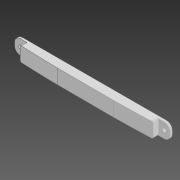
# Autodesk Inventor part: MidiPickup
Saved by Autodesk Inventor 2020 (Build 240168000, 168)
## iProperties
Created: 2022-11-12
Part Number: MidiPickup
Material: Generic
Document SubType Name: Modeling
Designer: valer
Density: 1 g/cm^3
Appearance: Default
Author: valer
Autodesk Inventor part; units mm, degrees
ref_plane "YZ Plane" through (0, 0, 0) normal (1, 0, 0) x (0, 1, 0)
ref_plane "XZ Plane" through (0, 0, 0) normal (0, 1, 0) x (-1, 0, 0)
ref_plane "XY Plane" through (0, 0, 0) normal (0, 0, 1) x (1, 0, 0)
sketch "Base" plane through (0, 0, 0) normal (0, 0, 1) x (1, 0, 0)
  line L0 (-64, -0.5) -> (64, -0.5) construction
  circle A0 centre (-64, -0.5) radius 1.5
  circle A1 centre (64, -0.5) radius 1.5
  line L1 (-64, 6) -> (64, 6)
  line L2 (69, 1) -> (69, -2)
  line L3 (64, -7) -> (-64, -7)
  line L4 (-69, -2) -> (-69, 1)
  line L5 (-59, 6) -> (-59, -7) construction
  line L6 (59, 6) -> (59, -7) construction
  arc A2 (-64, 6) -> (-69, 1) centre (-64, 1) ccw
  arc A3 (-69, -2) -> (-64, -7) centre (-64, -2) ccw
  arc A4 (69, 1) -> (64, 6) centre (64, 1) ccw
  arc A5 (64, -7) -> (69, -2) centre (64, -2) ccw
  point P0 (0, 0)
  dimension "d0" = 128
  dimension "d1" = 3
  dimension "d2" = 3
  dimension "d3" = 5
  dimension "d4" = 5
  dimension "d5" = 5
  dimension "d6" = 5
  dimension "d7" = 5
  dimension "d8" = 6.5
  dimension "d9" = 6.5
  constraints: 14 end point, 8 point on circle, 8 tangent, 6 centre point, 4 point on line, 3 equal radius, 2 coincident, 2 horizontal, 2 parallel, 2 vertical, 1 perpendicular
  measures "d0" distance of L0.start L0.end
  measures "d1" diameter of A0
  measures "d2" diameter of A1
  measures "d3" distance from line of L4 L0.start
  measures "d4" distance from line of L2 L0.end
  measures "d5" distance from line of L0.start L5
  measures "d6" distance from line of L0.end L6
  measures "d7" radius of A2
  measures "d8" distance between parallel lines of L1 L0
  measures "d9" distance between parallel lines of L3 L0
extrude "BaseFeature" add sketch "Base" along normal blind 2
sketch "Sketch2" plane through (0, 0, 2) normal (0, 0, 1) x (1, 0, 0)
  line L0 (-59, 6) -> (-59, -7) construction
  line L1 (59, 6) -> (59, -7) construction
  line L2 (58, 6) -> (-58, 6)
  line L3 (64, 6) -> (-64, 6) construction
  line L4 (-59, 5) -> (-59, -6)
  line L5 (-58, -7) -> (58, -7)
  line L6 (59, -6) -> (59, 5)
  arc A0 (-58, 6) -> (-59, 5) centre (-58, 5) ccw
  arc A1 (-59, -6) -> (-58, -7) centre (-58, -6) ccw
  arc A2 (59, 5) -> (58, 6) centre (58, 5) ccw
  arc A3 (58, -7) -> (59, -6) centre (58, -6) ccw
  point P0 (0, 0)
  dimension "d12" = 1
  dimension "d13" = 1
  constraints: 8 end point, 8 point on circle, 8 point on line, 8 tangent, 4 centre point, 3 collinear, 2 equal radius, 1 perpendicular
  measures "d12" radius of A0
  measures "d13" radius of A1
extrude "Extrusion2" add sketch "Sketch2" along normal blind 6
sketch "Sketch3" plane through (-64, -7, 0) normal (0, -1, 0) x (1, 0, 0)
  line L0 (0, 0) -> (128, 0) construction
  line L1 (128, 0) -> (128, 2) construction
  line L2 (122, 2) -> (128, 2) construction
  line L3 (6, 8) -> (122, 8) construction
  line L4 (0, 2) -> (6, 2) construction
  line L5 (0, 0) -> (0, 2) construction
  line L6 (64, 0) -> (64, 8.0447) construction
  line L7 (6, 8) -> (122, 8) construction
  arc A0 (64, 8.0447) -> (5, 7) centre (53.5583, -1068.8352) ccw
  arc A1 (123, 7) -> (64, 8.0447) centre (74.4417, -1068.8352) ccw
  line L8 (5, 2) -> (5, 8) projected
  line L9 (123, 2) -> (123, 8) projected
  line L10 (123, 8) -> (5, 8)
  point P0 (88.7678, 8)
  point P1 (39.2322, 8)
  dimension "d17" = 1076.9305
  dimension "d22" = 1
  dimension "d23" = 1
  constraints: 4 end point, 4 point on circle, 2 centre point, 2 perpendicular, 2 point on line, 1 symmetric about line, 2 other
  measures "d17" radius of A1
  measures "d22" distance of L8.end A0.end
  measures "d23" distance of L9.end A1.start
extrude "Extrusion4" cut sketch "Sketch3" against normal through all contours L10 L9 A1 | A0 L8 L10
equation "\"d9\" = d8"
body "Solid1"
